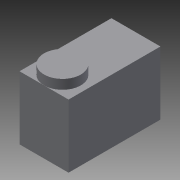
# Autodesk Inventor part: herkulex
Saved by Autodesk Inventor 2015 (Build 190159000, 159)
## iProperties
Created: 2014-10-18
Part Number: herkulex
Material: Generic
Document SubType Name: Modeling
Designer: ericd_000
Density: 1 g/cm^3
Appearance: Default
Author: ericd_000
Autodesk Inventor part; units mm, degrees
ref_plane "YZ Plane" through (0, 0, 0) normal (1, 0, 0) x (0, 1, 0)
ref_plane "XZ Plane" through (0, 0, 0) normal (0, 1, 0) x (-1, 0, 0)
ref_plane "XY Plane" through (0, 0, 0) normal (0, 0, 1) x (1, 0, 0)
sketch "Sketch1" plane through (0, 0, 0) normal (0, 0, 1) x (1, 0, 0)
  line L0 (-12, 22.5) -> (12, 22.5)
  line L1 (12, 22.5) -> (12, -22.5)
  line L2 (12, -22.5) -> (-12, -22.5)
  line L3 (-12, -22.5) -> (-12, 22.5)
  point P0 (0, 0)
  point P1 (12, 0)
  point P2 (0, 22.5)
  dimension "d0" = 24
  dimension "d1" = 45
  constraints: 8 end point, 2 midpoint, 2 parallel, 1 horizontal, 1 horizontal alignment, 1 perpendicular, 1 vertical alignment
  measures "d0" distance of L0.start L0.end
  measures "d1" distance of L2.end L0.start
extrude "Extrusion1" add sketch "Sketch1" along normal blind 31
sketch "Sketch2" plane through (0, 0, 31) normal (0, 0, 1) x (1, 0, 0)
  circle A0 centre (0, -13.5) radius 9
  line L0 (-12, -22.5) -> (12, -22.5) projected
  point P0 (0, 0)
  dimension "d4" = 18
  constraints: 1 centre point, 1 tangent
  measures "d4" diameter of A0
extrude "Extrusion2" add sketch "Sketch2" along normal blind 4.6
body "Solid1"
